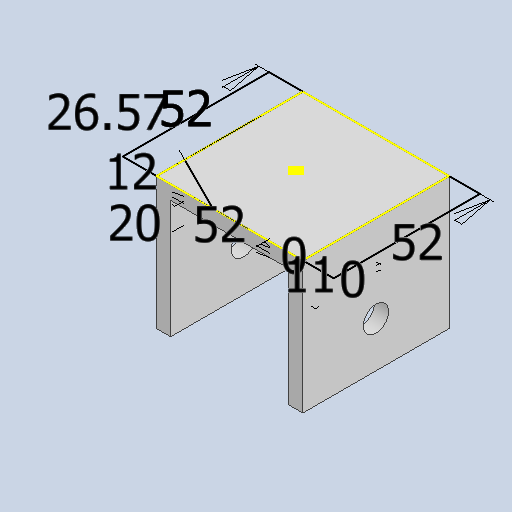
# Autodesk Inventor part: new_camera_case_front
Saved by Autodesk Inventor 2025.2 (Build 292293000, 293)
## iProperties
Created: 2025-05-20
Part Number: new_camera_case_front
Material: 일반
Document SubType Name: Modeling
Designer: jbhma
Density: 1 g/cm^3
Appearance: 기본값
Author: jbhma
Autodesk Inventor part; units mm, degrees
ref_plane "YZ Plane" through (0, 0, 0) normal (1, 0, 0) x (0, 1, 0)
ref_plane "XZ Plane" through (0, 0, 0) normal (0, 1, 0) x (-1, 0, 0)
ref_plane "XY Plane" through (0, 0, 0) normal (0, 0, 1) x (1, 0, 0)
sketch "스케치1" plane through (0, 0, 0) normal (0, 1, 0) x (-1, 0, 0)
  line L0 (24.089, 25.4241) -> (-27.911, 25.4241)
  line L1 (-27.911, 25.4241) -> (-27.911, -26.5759)
  line L2 (-27.911, -26.5759) -> (24.089, -26.5759)
  line L3 (24.089, -26.5759) -> (24.089, 25.4241)
  point P0 (0, 0)
  dimension "d0" = 52
  dimension "d1" = 52
  constraints: 8 end point, 2 parallel, 1 coincident, 1 horizontal, 1 perpendicular
  measures "d0" distance of L2.end L1.end
  measures "d1" distance of L1.end L0.end
extrude "돌출2" add sketch "스케치1" along normal blind 5
sketch "스케치2" plane through (0, 0, 0) normal (0, -1, 0) x (1, 0, 0)
  line L0 (27.911, 25.4241) -> (27.911, -26.5759) projected
  line L1 (-24.089, 25.4241) -> (27.911, 25.4241) projected
  line L2 (-24.089, -26.5759) -> (-24.089, 25.4241) projected
  line L3 (27.911, -26.5759) -> (-24.089, -26.5759) projected
  line L4 (-24.089, 25.4241) -> (-19.089, 25.4241)
  line L5 (-19.089, 25.4241) -> (-19.089, -26.5759)
  line L6 (-19.089, -26.5759) -> (-24.089, -26.5759)
  line L7 (-24.089, -26.5759) -> (-24.089, 25.4241)
  line L8 (27.911, 25.4241) -> (22.911, 25.4241)
  line L9 (22.911, 25.4241) -> (22.911, -26.5759)
  line L10 (22.911, -26.5759) -> (27.911, -26.5759)
  line L11 (27.911, -26.5759) -> (27.911, 25.4241)
  point P0 (0, 0)
  dimension "d8" = 5
  dimension "d9" = 5
  constraints: 16 end point, 4 parallel, 2 horizontal, 2 perpendicular, 2 point on line
  measures "d8" distance of L5.end L6.end
  measures "d9" distance of L10.end L9.end
extrude "돌출3" add sketch "스케치2" along normal blind 42 contours L0 L3 L9 L1 | L5 L3 L2 L1
sketch "스케치4" plane through (0, 5, 0) normal (0, 1, 0) x (1, 0, 0)
  line L0 (27.911, -25.4241) -> (27.911, 26.5759) projected
  line L1 (27.911, 26.5759) -> (-24.089, 26.5759) projected
  line L2 (-24.089, 26.5759) -> (-24.089, -25.4241) projected
  line L3 (-24.089, -25.4241) -> (27.911, -25.4241) projected
  line L4 (27.911, 26.5759) -> (38.911, 26.5759)
  line L5 (38.911, 26.5759) -> (38.911, -25.4241)
  line L6 (38.911, -25.4241) -> (27.911, -25.4241)
  line L7 (27.911, -25.4241) -> (27.911, 26.5759)
  line L8 (-24.089, 26.5759) -> (-36.089, 26.5759)
  line L9 (-36.089, 26.5759) -> (-36.089, -25.4241)
  line L10 (-36.089, -25.4241) -> (-24.089, -25.4241)
  line L11 (-24.089, -25.4241) -> (-24.089, 26.5759)
  line L12 (-24.089, 26.5759) -> (27.911, 26.5759)
  line L13 (27.911, 26.5759) -> (27.911, -25.4241)
  line L14 (27.911, -25.4241) -> (-24.089, -25.4241)
  line L15 (-24.089, -25.4241) -> (-24.089, 26.5759)
  line L16 (-24.089, -15.4219) -> (-4.089, -25.4241)
  point P0 (0, 0)
  point P1 (-24.089, -25.4241)
  dimension "d12" = 11
  dimension "d13" = 12
  dimension "d32" = 0
  dimension "d33" = 52
  dimension "d34" = 52
  dimension "d35" = 0
  dimension "d36" = 52
  dimension "d37" = 52
  dimension "d38" = 26.57
  dimension "d39" = 20
  constraints: 26 end point, 6 parallel, 3 horizontal, 3 perpendicular, 2 point on line
  measures "d12" distance of L5.end L6.end
  measures "d13" distance of L10.end L9.end
  measures "d32" distance between parallel lines of L3 L6
  measures "d33" distance between parallel lines of L1 L10
  measures "d34" distance from line of point (27.911, -25.424) L1
  measures "d35" distance from line of point (27.911, -25.424) L0
  measures "d36" distance from line of point (-24.089, -25.424) L1
  measures "d37" distance from line of point (-24.089, -25.424) L0
  measures "d38" angle of L3 L16
  measures "d39" distance from line of L16.end L11
sketch "스케치8" plane through (27.911, -42, 25.4241) normal (1, 0, 0) x (0, 0, -1)
  line L0 (52, 0) -> (52, 47) projected
  line L1 (0, 47) -> (52, 47) projected
  line L2 (0, 47) -> (0, 0) projected
  line L3 (52, 0) -> (0, 0) projected
  circle A0 centre (26, 16.074) radius 4.5
  point P0 (25.4241, 42)
  point P1 (26, 0)
  dimension "d26" = 9
  dimension "d27" = 16.074
  constraints: 1 centre point, 1 midpoint, 1 vertical alignment
  measures "d26" diameter of A0
  measures "d27" distance from line of L3 A0.centre
extrude "돌출8" cut sketch "스케치8" along normal mid plane 150 contours A0
